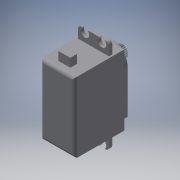
# Autodesk Inventor part: Base
Saved by Autodesk Inventor 2017 (Build 210142000, 142)
## iProperties
Part Number: Base
Material: Genérico
Document SubType Name: Modeling
Designer: Daniel Caycedo
Density: 1 g/cm^3
Appearance: Valor por defecto
Author: Daniel Caycedo
Autodesk Inventor part; units mm, degrees
ref_plane "YZ Plane" through (0, 0, 0) normal (1, 0, 0) x (0, 1, 0)
ref_plane "XZ Plane" through (0, 0, 0) normal (0, 1, 0) x (-1, 0, 0)
ref_plane "XY Plane" through (0, 0, 0) normal (0, 0, 1) x (1, 0, 0)
sketch "Boceto1" plane through (0, 0, 0) normal (0, 1, 0) x (-1, 0, 0)
  line L0 (10, 20.5) -> (-10, 20.5)
  line L1 (-10, 20.5) -> (-10, -20.5)
  line L2 (-10, -20.5) -> (10, -20.5)
  line L3 (10, -20.5) -> (10, 20.5)
  line L4 (10, 20.5) -> (-10, -20.5) construction
  line L5 (-10, 20.5) -> (10, -20.5) construction
  point P0 (0, 0)
  dimension "d0" = 20
  dimension "d1" = 41
  constraints: 12 end point, 2 midpoint, 2 parallel, 1 horizontal, 1 perpendicular
  measures "d0" distance of L2.end L1.end
  measures "d1" distance of L1.end L0.end
extrude "Extrusión1" add sketch "Boceto1" along normal blind 21
sketch "Boceto2" plane through (0, 21, 0) normal (0, 1, 0) x (1, 0, 0)
  line L0 (-9, -27.5) -> (9, -27.5)
  line L1 (9, -27.5) -> (9, 27.5)
  line L2 (9, 27.5) -> (-9, 27.5)
  line L3 (-9, 27.5) -> (-9, -27.5)
  line L4 (-9, -27.5) -> (9, 27.5) construction
  line L5 (9, -27.5) -> (-9, 27.5) construction
  point P0 (0, 0)
  dimension "d4" = 18
  dimension "d5" = 55
  constraints: 12 end point, 2 midpoint, 2 parallel, 1 horizontal, 1 perpendicular
  measures "d4" distance of L2.end L1.end
  measures "d5" distance of L1.end L0.end
extrude "Extrusión2" add sketch "Boceto2" along normal blind 2
sketch "Boceto3" plane through (0, 21, 0) normal (0, 1, 0) x (1, 0, 0)
  line L0 (-10, -20.5) -> (10, -20.5) projected
  line L1 (10, -20.5) -> (-10, -20.5)
  line L2 (-10, -20.5) -> (-10, 20.5)
  line L3 (-10, 20.5) -> (10, 20.5)
  line L4 (10, 20.5) -> (10, -20.5)
  point P0 (0, 0)
  constraints: 8 end point, 2 parallel, 1 horizontal, 1 perpendicular
extrude "Extrusión3" add sketch "Boceto3" along normal blind 2
sketch "Boceto4" plane through (0, 23, 0) normal (0, 1, 0) x (1, 0, 0)
  line L0 (-10, 20.5) -> (-10, -20.5) projected
  line L1 (10, -20.5) -> (-10, -20.5)
  line L2 (-10, -20.5) -> (-10, 20.5)
  line L3 (-10, 20.5) -> (10, 20.5)
  line L4 (10, 20.5) -> (10, -20.5)
  line L5 (10, -20.5) -> (-10, 20.5) construction
  line L6 (-10, -20.5) -> (10, 20.5) construction
  point P0 (0, 0)
  constraints: 12 end point, 2 midpoint, 2 parallel, 1 horizontal, 1 perpendicular
extrude "Extrusión4" add sketch "Boceto4" along normal blind 6
fillet "Empalme1" radius 2 4 edges at (0, 0, 20.5) (-10, 0, 0) (10, 0, 0) (0, 0, -20.5)
sketch "Boceto5" plane through (-10, 29, 20.5) normal (0, 0, 1) x (1, 0, 0)
  line L0 (10, -29) -> (10, -25)
  line L1 (10, -25) -> (10, -23)
  line L2 (13.5, -21) -> (6.5, -21)
  line L3 (6.5, -21) -> (6.5, -25)
  line L4 (6.5, -25) -> (13.5, -25)
  line L5 (13.5, -25) -> (13.5, -21)
  line L6 (13.5, -21) -> (6.5, -25) construction
  line L7 (6.5, -21) -> (13.5, -25) construction
  dimension "d13" = 4
  dimension "d14" = 2
  dimension "d15" = 7
  dimension "d16" = 4
  constraints: 16 end point, 2 midpoint, 2 parallel, 1 horizontal, 1 perpendicular, 1 point on line, 1 vertical
  measures "d13" distance of L0.start L0.end
  measures "d14" distance of L0.end L1.end
  measures "d15" distance of L4.end L3.end
  measures "d16" distance of L3.end L2.end
extrude "Extrusión5" add sketch "Boceto5" along normal blind 5
fillet "Empalme2" radius 2 4 edges at (-9, 22, 27.5) (9, 22, 27.5) (-9, 22, -27.5) (9, 22, -27.5)
sketch "Boceto6" plane through (0, 23, 0) normal (0, 1, 0) x (1, 0, 0)
  line L0 (9, -25.5) -> (9, -20.5) projected
  arc A0 (7, -27.5) -> (9, -25.5) centre (7, -25.5) ccw projected
  line L1 (9, -25.5) -> (7, -25.5)
  line L2 (7, -25.5) -> (7, -27.5)
  line L3 (7, -27.5) -> (9, -27.5)
  line L4 (9, -27.5) -> (9, -25.5)
  line L5 (9, -27.5) -> (5, -27.5)
  line L6 (5, -27.5) -> (5, -25.5)
  line L7 (5, -25.5) -> (9, -25.5)
  line L8 (9, -25.5) -> (9, -27.5)
  circle A1 centre (5, -25.5) radius 2.5
  line L9 (-7, -27.5) -> (7, -27.5) projected
  line L10 (0, -27.5) -> (0, 27.5)
  line L11 (7, 27.5) -> (-7, 27.5) projected
  line L12 (10, 20.5) -> (10, -20.5) projected
  line L13 (10, 0) -> (-10, 0)
  line L14 (-10, -20.5) -> (-10, 20.5) projected
  circle A2 centre (-5, -25.5) radius 2.5
  line L15 (-10, 0) -> (10, 0)
  circle A3 centre (5, 25.5) radius 2.5
  circle A4 centre (-5, 25.5) radius 2.5
  point P0 (0, 0)
  dimension "d20" = 4
  dimension "d21" = 2
  dimension "d22" = 5
  constraints: 22 end point, 5 symmetric about line, 4 centre point, 4 midpoint, 4 parallel, 2 horizontal, 2 perpendicular, 1 coincident, 3 other
  measures "d20" distance of L6.end L7.end
  measures "d21" distance of L5.end L6.end
  measures "d22" diameter of A1
extrude "Extrusión6" cut sketch "Boceto6" against normal blind 2 contours A2 L9 | L9 A2 | A4 L11 | L11 A4 | A3 L11 | L11 A3 | A1 L5 L6 L7 L2 | L2 L1 A1 | A1 L9 L5 | L1 L7 L6 L9 A1
sketch "Boceto7" plane through (0, 29, 0) normal (0, 1, 0) x (1, 0, 0)
  line L0 (10, 20.5) -> (-10, 20.5) projected
  line L1 (-10, 20.5) -> (10, 20.5)
  line L2 (10, -20.5) -> (10, 20.5) projected
  line L3 (10, 14.5) -> (10, -10.5)
  line L4 (-10, -20.5) -> (10, -20.5) projected
  line L5 (-10, -20.5) -> (-10, 14.5)
  circle A0 centre (0, -10.5) radius 10
  line L6 (10, 20.5) -> (10, 14.5)
  line L7 (10, 14.5) -> (-10, 14.5)
  circle A1 centre (0, 14.5) radius 2.5
  point P0 (0, 0)
  dimension "d25" = 6
  dimension "d26" = 90
  dimension "d27" = 5
  constraints: 10 end point, 2 collinear, 2 vertical, 1 centre point, 1 horizontal, 1 horizontal alignment, 1 midpoint, 2 other
  measures "d25" distance of L3.start L0.start
  measures "d26" angle of L6 L7
  measures "d27" diameter of A1
extrude "Extrusión7" add sketch "Boceto7" along normal blind 2 contours A0 | A1 L7 | L7 A1
sketch "Boceto8" plane through (0, 29, 0) normal (0, 1, 0) x (1, 0, 0)
  circle A0 centre (0, -10.5) radius 10 projected
  circle A1 centre (0, 14.5) radius 2.5 projected
  line L0 (0, -10.5) -> (0, 14.5)
  line L1 (10, -10.5) -> (10, 20.5) projected
  line L2 (-10, -10.5) -> (10, -10.5)
  line L3 (10, -10.5) -> (10, 14.5)
  line L4 (10, 14.5) -> (-10, 14.5)
  line L5 (-10, 14.5) -> (-10, -10.5)
  line L6 (-10, -10.5) -> (10, 14.5) construction
  line L7 (10, -10.5) -> (-10, 14.5) construction
  point P0 (0, 0)
  point P1 (0, 2)
  constraints: 14 end point, 3 midpoint, 2 parallel, 1 horizontal, 1 horizontal alignment, 1 perpendicular, 1 point on line, 1 vertical
extrude "Extrusión8" add sketch "Boceto8" along normal blind 2 contours L5 L4 A1 L0 A0 | A0 L0 L2 | L2 L0 A0 | A0 L0 A1 L4 L1 | L0 L4 A1 | A1 L4 L0
sketch "Boceto9" plane through (0, 31, 0) normal (0, 1, 0) x (1, 0, 0)
  arc A0 (0, -20.5) -> (10, -10.5) centre (0, -10.5) ccw projected
  circle A1 centre (0, -10.5) radius 6.5
  point P0 (0, 0)
  dimension "d32" = 13
  constraints: 1 centre point, 1 coincident
  measures "d32" diameter of A1
extrude "Extrusión9" add sketch "Boceto9" along normal blind 2
sketch "Boceto10" plane through (0, 33, 10.5) normal (0, 1, 0) x (1, 0, 0)
  circle A0 centre (0, 0) radius 6.5 projected
  circle A1 centre (0, 0) radius 3
  point P0 (0, 10.5)
  dimension "d35" = 6
  constraints: 1 centre point, 1 coincident
  measures "d35" diameter of A1
extrude "Extrusión10" add sketch "Boceto10" along normal blind 5 contours A1
sketch "Boceto11" plane through (0, 38, 10.5) normal (0, 1, 0) x (1, 0, 0)
  circle A0 centre (0, 0) radius 3 projected
  line L0 (0, 0) -> (0, 3)
  line L1 (0, 3) -> (0, 2.8)
  line L2 (-0.3464, 2.8) -> (0, 3.4)
  line L3 (0, 3.4) -> (0.3464, 2.8)
  line L4 (0.3464, 2.8) -> (-0.3464, 2.8)
  line L5 (-1.0593, 2.6149) -> (-0.88, 3.2841)
  line L6 (-0.88, 3.2841) -> (-0.3901, 2.7942)
  line L7 (-0.3901, 2.7942) -> (-1.0593, 2.6149)
  line L8 (-1.7, 2.2517) -> (-1.7, 2.9445)
  line L9 (-1.7, 2.9445) -> (-1.1, 2.5981)
  line L10 (-1.1, 2.5981) -> (-1.7, 2.2517)
  line L11 (-2.2248, 1.735) -> (-2.4042, 2.4042)
  line L12 (-2.4042, 2.4042) -> (-1.735, 2.2248)
  line L13 (-1.735, 2.2248) -> (-2.2248, 1.735)
  line L14 (-2.5981, 1.1) -> (-2.9445, 1.7)
  line L15 (-2.9445, 1.7) -> (-2.2517, 1.7)
  line L16 (-2.2517, 1.7) -> (-2.5981, 1.1)
  line L17 (-2.7942, 0.3901) -> (-3.2841, 0.88)
  line L18 (-3.2841, 0.88) -> (-2.6149, 1.0593)
  line L19 (-2.6149, 1.0593) -> (-2.7942, 0.3901)
  line L20 (-2.8, -0.3464) -> (-3.4, 0)
  line L21 (-3.4, 0) -> (-2.8, 0.3464)
  line L22 (-2.8, 0.3464) -> (-2.8, -0.3464)
  line L23 (-2.6149, -1.0593) -> (-3.2841, -0.88)
  line L24 (-3.2841, -0.88) -> (-2.7942, -0.3901)
  line L25 (-2.7942, -0.3901) -> (-2.6149, -1.0593)
  line L26 (-2.2517, -1.7) -> (-2.9445, -1.7)
  line L27 (-2.9445, -1.7) -> (-2.5981, -1.1)
  line L28 (-2.5981, -1.1) -> (-2.2517, -1.7)
  line L29 (-1.735, -2.2248) -> (-2.4042, -2.4042)
  line L30 (-2.4042, -2.4042) -> (-2.2248, -1.735)
  line L31 (-2.2248, -1.735) -> (-1.735, -2.2248)
  line L32 (-1.1, -2.5981) -> (-1.7, -2.9445)
  line L33 (-1.7, -2.9445) -> (-1.7, -2.2517)
  line L34 (-1.7, -2.2517) -> (-1.1, -2.5981)
  line L35 (-0.3901, -2.7942) -> (-0.88, -3.2841)
  line L36 (-0.88, -3.2841) -> (-1.0593, -2.6149)
  line L37 (-1.0593, -2.6149) -> (-0.3901, -2.7942)
  line L38 (0.3464, -2.8) -> (0, -3.4)
  line L39 (0, -3.4) -> (-0.3464, -2.8)
  line L40 (-0.3464, -2.8) -> (0.3464, -2.8)
  line L41 (1.0593, -2.6149) -> (0.88, -3.2841)
  line L42 (0.88, -3.2841) -> (0.3901, -2.7942)
  line L43 (0.3901, -2.7942) -> (1.0593, -2.6149)
  line L44 (1.7, -2.2517) -> (1.7, -2.9445)
  line L45 (1.7, -2.9445) -> (1.1, -2.5981)
  line L46 (1.1, -2.5981) -> (1.7, -2.2517)
  line L47 (2.2248, -1.735) -> (2.4042, -2.4042)
  line L48 (2.4042, -2.4042) -> (1.735, -2.2248)
  line L49 (1.735, -2.2248) -> (2.2248, -1.735)
  line L50 (2.5981, -1.1) -> (2.9445, -1.7)
  line L51 (2.9445, -1.7) -> (2.2517, -1.7)
  line L52 (2.2517, -1.7) -> (2.5981, -1.1)
  line L53 (2.7942, -0.3901) -> (3.2841, -0.88)
  line L54 (3.2841, -0.88) -> (2.6149, -1.0593)
  line L55 (2.6149, -1.0593) -> (2.7942, -0.3901)
  line L56 (2.8, 0.3464) -> (3.4, 0)
  line L57 (3.4, 0) -> (2.8, -0.3464)
  line L58 (2.8, -0.3464) -> (2.8, 0.3464)
  line L59 (2.6149, 1.0593) -> (3.2841, 0.88)
  line L60 (3.2841, 0.88) -> (2.7942, 0.3901)
  line L61 (2.7942, 0.3901) -> (2.6149, 1.0593)
  line L62 (2.2517, 1.7) -> (2.9445, 1.7)
  line L63 (2.9445, 1.7) -> (2.5981, 1.1)
  line L64 (2.5981, 1.1) -> (2.2517, 1.7)
  line L65 (1.735, 2.2248) -> (2.4042, 2.4042)
  line L66 (2.4042, 2.4042) -> (2.2248, 1.735)
  line L67 (2.2248, 1.735) -> (1.735, 2.2248)
  line L68 (1.1, 2.5981) -> (1.7, 2.9445)
  line L69 (1.7, 2.9445) -> (1.7, 2.2517)
  line L70 (1.7, 2.2517) -> (1.1, 2.5981)
  line L71 (0.3901, 2.7942) -> (0.88, 3.2841)
  line L72 (0.88, 3.2841) -> (1.0593, 2.6149)
  line L73 (1.0593, 2.6149) -> (0.3901, 2.7942)
  point P0 (0, 10.5)
  point P1 (-0.7247, 2.7046)
  point P2 (-1.4, 2.4249)
  point P3 (-1.9799, 1.9799)
  point P4 (-2.4249, 1.4)
  point P5 (-2.7046, 0.7247)
  point P6 (-2.8, 0)
  point P7 (-2.7046, -0.7247)
  point P8 (-2.4249, -1.4)
  point P9 (-1.9799, -1.9799)
  point P10 (-1.4, -2.4249)
  point P11 (-0.7247, -2.7046)
  point P12 (0, -2.8)
  point P13 (0.7247, -2.7046)
  point P14 (1.4, -2.4249)
  point P15 (1.9799, -1.9799)
  point P16 (2.4249, -1.4)
  point P17 (2.7046, -0.7247)
  point P18 (2.8, 0)
  point P19 (2.7046, 0.7247)
  point P20 (2.4249, 1.4)
  point P21 (1.9799, 1.9799)
  point P22 (1.4, 2.4249)
  point P23 (0.7247, 2.7046)
  dimension "d38" = 0.2
  dimension "d41" = 360
  constraints: 148 end point, 1 coincident, 1 midpoint, 1 point on line, 1 vertical, 1 vertical alignment, 177 other
  measures "d38" distance of L0.end L1.end
extrude "Extrusión11" add sketch "Boceto11" against normal blind 5
